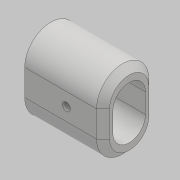
# Autodesk Inventor part: exercise3-8
Saved by Autodesk Inventor 2018 (Build 220112000, 112)
## iProperties
Created: 2020-09-23
Part Number: exercise3-8
Material: 一般
Document SubType Name: Modeling
Designer: 王鼎鈞
Density: 1 g/cm^3
Appearance: 預設
Author: 王鼎鈞
Autodesk Inventor part; units mm, degrees
ref_plane "YZ Plane" through (0, 0, 0) normal (1, 0, 0) x (0, 1, 0)
ref_plane "XZ Plane" through (0, 0, 0) normal (0, 1, 0) x (-1, 0, 0)
ref_plane "XY Plane" through (0, 0, 0) normal (0, 0, 1) x (1, 0, 0)
sketch "草圖1" plane through (0, 0, 0) normal (1, 0, 0) x (0, 1, 0)
  line L0 (-20, 30) -> (20, 30)
  line L1 (20, 30) -> (20, -30)
  line L2 (20, -30) -> (-20, -30)
  line L3 (-20, -30) -> (-20, 30)
  line L4 (-20, 30) -> (20, -30) construction
  line L5 (20, 30) -> (-20, -30) construction
  line L6 (-12.5, 20) -> (12.5, 20)
  line L7 (12.5, 20) -> (12.5, -20)
  line L8 (12.5, -20) -> (-12.5, -20)
  line L9 (-12.5, -20) -> (-12.5, 20)
  line L10 (-12.5, 20) -> (12.5, -20) construction
  line L11 (12.5, 20) -> (-12.5, -20) construction
  point P0 (0, 0)
  dimension "d0" = 40
  dimension "d1" = 60
  dimension "d2" = 25
  dimension "d3" = 40
  constraints: 24 end point, 4 midpoint, 4 parallel, 2 horizontal, 2 perpendicular
  measures "d0" distance of L1.end L2.end
  measures "d1" distance of L0.end L1.end
  measures "d2" distance of L7.end L8.end
  measures "d3" distance of L6.end L7.end
extrude "擠出1" add sketch "草圖1" along normal blind 60
fillet "圓角1" radius 20 4 edges at (30, 20, 30) (30, -20, 30) (30, 20, -30) (30, -20, -30)
fillet "圓角2" radius 12.5 4 edges at (30, 12.5, 20) (30, -12.5, 20) (30, -12.5, -20) (30, 12.5, -20)
chamfer "倒角1" distance 5 angle 45 4 edges at (60, 14.1422, -24.1422) (60, -20, 0) (60, 14.1422, 24.1422) (60, 20, 0)
sketch "草圖2" plane through (0, -20, -10) normal (0, -1, 0) x (1, 0, 0)
  line L0 (-12, 10) -> (72, 10) projected
  line L1 (0, -32) -> (0, 52) projected
  line L2 (60, 0) -> (60, 20) projected
  line L3 (32, 0) -> (32, 20)
  circle A0 centre (32, 10) radius 3
  point P0 (0, 10)
  dimension "d11" = 28
  dimension "d12" = 6
  constraints: 2 end point, 1 centre point, 1 midpoint, 1 parallel
  measures "d11" distance between parallel lines of L2 L3
  measures "d12" diameter of A0
extrude "擠出2" cut sketch "草圖2" against normal blind 157.75
